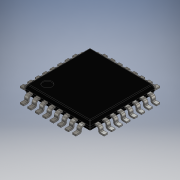
# Autodesk Inventor part: 32 TQFP
Saved by Autodesk Inventor 2016 (Build 200138000, 138)
## iProperties
Created: 2016-07-01
Part Number: 32 TQFP
Material: Generic
Document SubType Name: Modeling
Designer: Jonathan
Density: 1 g/cm^3
Appearance: Default
Author: Jonathan
Autodesk Inventor part; units mm, degrees
ref_plane "YZ Plane" through (0, 0, 0) normal (1, 0, 0) x (0, 1, 0)
ref_plane "XZ Plane" through (0, 0, 0) normal (0, 1, 0) x (-1, 0, 0)
ref_plane "XY Plane" through (0, 0, 0) normal (0, 0, 1) x (1, 0, 0)
sketch "Sketch1" plane through (0, 0, 0) normal (0, 1, 0) x (-1, 0, 0)
  line L0 (3.5, 3.5) -> (-3.5, 3.5)
  line L1 (-3.5, 3.5) -> (-3.5, -3.5)
  line L2 (-3.5, -3.5) -> (3.5, -3.5)
  line L3 (3.5, -3.5) -> (3.5, 3.5)
  point P0 (0, 0)
  point P1 (3.5, 0)
  point P2 (0, -3.5)
  dimension "d0" = 7
  dimension "d1" = 7
  constraints: 8 end point, 2 midpoint, 2 parallel, 1 horizontal, 1 horizontal alignment, 1 perpendicular, 1 vertical alignment
  measures "d0" distance of L1.end L2.end
  measures "d1" distance of L0.end L1.end
extrude "Extrusion1" add sketch "Sketch1" along normal blind 1
ref_plane "Work Plane1" through (2.8, 0, 3.5) normal (1, 0, 0) x (0, 0, -1)
sketch "Sketch2" plane through (2.8, 0, 3.5) normal (1, 0, 0) x (0, 0, -1)
  line L0 (7.175, 0.575) -> (7, 0.575)
  line L1 (7, 0.575) -> (7, 0.425)
  line L2 (7, 0.425) -> (7.175, 0.425)
  line L3 (7.3875, 0.2125) -> (7.3875, 0.1125)
  line L4 (7.5375, 0.2125) -> (7.5375, 0.1125)
  line L5 (7.6, 0.05) -> (8, 0.05)
  line L6 (8, 0.05) -> (8, -0.1)
  line L7 (8, -0.1) -> (7.6, -0.1)
  arc A0 (7.5375, 0.2125) -> (7.175, 0.575) centre (7.175, 0.2125) ccw
  arc A1 (7.3875, 0.2125) -> (7.175, 0.425) centre (7.175, 0.2125) ccw
  arc A2 (7.5375, 0.1125) -> (7.6, 0.05) centre (7.6, 0.1125) ccw
  arc A3 (7.3875, 0.1125) -> (7.6, -0.1) centre (7.6, 0.1125) ccw
  line L8 (7, 0) -> (7, 1) projected
  line L9 (0, 0) -> (7, 0) projected
  point P0 (3.5, 0)
  point P1 (7, 0.5)
  dimension "d5" = 0.15
  dimension "d6" = 0.1
  dimension "d7" = 1
  dimension "d8" = 0.1
  dimension "d9" = 0.4
  constraints: 16 end point, 8 point on circle, 8 tangent, 4 centre point, 4 perpendicular, 2 concentric, 2 horizontal, 2 midpoint, 2 vertical, 1 collinear, 1 equal radius
  measures "d5" distance of L0.end L1.end
  measures "d6" distance between parallel lines of L9 L7
  measures "d7" distance between parallel lines of L6 L8
  measures "d8" distance of L4.start L4.end
  measures "d9" distance of L6.end L7.end
extrude "Extrusion2" add sketch "Sketch2" along normal mid plane 0.375 separate body
pattern_linear "Rectangular Pattern1" count 8 spacing 0.8 along (-1, 0, 0) of "Extrusion2" bodies 2
pattern_circular "Circular Pattern1" count 4 over 360 about axis through (0, -10, 0) along (0, 1, 0) of "Extrusion2", "Rectangular Pattern1" bodies 2
chamfer "Chamfer1" distance 0.15 distance2 0.4 1 edges at (3.5, 1, 0) measured on face at (3, 1, 0)
chamfer "Chamfer2" distance 0.4 distance2 0.15 1 edges at (3.5, 0, 0) measured on face at (3.5, 0.1, 0)
chamfer "Chamfer3" distance 0.4 distance2 0.15 1 edges at (-0.075, 1, -3.5) measured on face at (-0.075, 0.5, -3.5)
chamfer "Chamfer4" distance 0.4 distance2 0.15 1 edges at (-0.075, 0, -3.5) measured on face at (-0.075, 0.1, -3.5)
chamfer "Chamfer5" distance 0.4 distance2 0.15 1 edges at (-3.5, 1, 0.075) measured on face at (-3.5, 0.5, 0.075)
chamfer "Chamfer6" distance 0.4 distance2 0.15 1 edges at (-3.5, 0, 0.075) measured on face at (-3.5, 0.1, 0.075)
chamfer "Chamfer7" distance 0.4 distance2 0.15 1 edges at (0, 1, 3.5) measured on face at (0, 0.5, 3.5)
chamfer "Chamfer8" distance 0.4 distance2 0.15 1 edges at (0, 0, 3.5) measured on face at (0, 0.1, 3.5)
fillet "Fillet2" radius 0.1 20 edges at (-3.425, 0.2, 3.425) (-3.5, 0.5, 3.5) (-3.425, 0.8, 3.425) (0, 1, 3.35) (-3.35, 1, 0) (-3.425, 0.8, -3.425) (-3.5, 0.5, -3.5) (-3.425, 0.2, -3.425) (0, 1, -3.35) (-3.35, 0, 0) (0, 0, -3.35) (3.425, 0.8, -3.425) (3.5, 0.5, -3.5) (3.425, 0.2, -3.425) (3.35, 1, 0) (3.35, 0, 0) (3.425, 0.8, 3.425) (3.5, 0.5, 3.5) (3.425, 0.2, 3.425) (0, 0, 3.35)
sketch "Sketch3" plane through (0, 1, 0) normal (0, 1, 0) x (1, 0, 0)
  circle A0 centre (-2.2807, 2.2807) radius 0.5
  line L0 (-3.2807, 3.2807) -> (3.2807, 3.2807) projected
  line L1 (-3.2807, -3.2807) -> (-3.2807, 3.2807) projected
  point P0 (0, 0)
  dimension "d44" = 1
  dimension "d45" = 1
  dimension "d46" = 1
  constraints: 1 centre point
  measures "d44" diameter of A0
  measures "d45" distance from line of A0.centre L0
  measures "d46" distance from line of L1 A0.centre
extrude "Extrusion3" cut sketch "Sketch3" against normal blind 0.1 bodies 1
body "Solid1"
body "Solid2"
